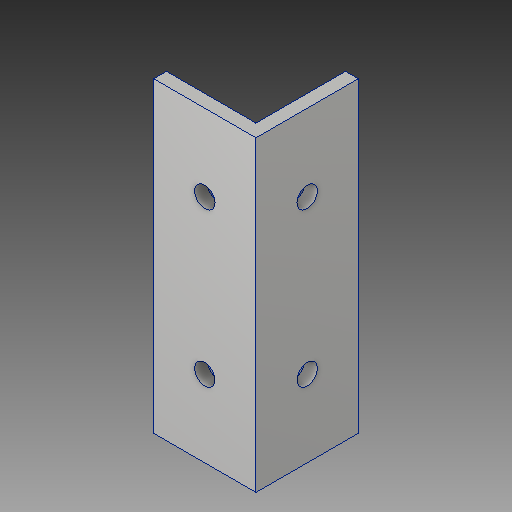
# Autodesk Inventor part: L Bracket 3in
Saved by Autodesk Inventor 2018 (Build 220112000, 112)
## iProperties
Created: 2018-01-19
Part Number: L Bracket 3in
Material: Aluminum 6061
Document SubType Name: Modeling
Designer: S-2512711
Density: 2.7 g/cm^3
Appearance: Aluminum - Flat
Mass: 30.4148 g
Surface Area: 80.8488 cm^2
Volume: 11.2647 cm^3
Author: S-2512711
Autodesk Inventor part; units mm, degrees
ref_plane "YZ Plane" through (0, 0, 0) normal (1, 0, 0) x (0, 1, 0)
ref_plane "XZ Plane" through (0, 0, 0) normal (0, 1, 0) x (-1, 0, 0)
ref_plane "XY Plane" through (0, 0, 0) normal (0, 0, 1) x (1, 0, 0)
sketch "Sketch1" plane through (0, 0, 0) normal (0, 1, 0) x (-1, 0, 0)
  line L0 (0, 0) -> (-25.4, 0)
  line L1 (-25.4, 0) -> (-25.4, -3.175)
  line L2 (-25.4, -3.175) -> (0, -3.175)
  line L3 (0, -3.175) -> (0, 0)
  line L4 (-25.4, 0) -> (-22.225, 0)
  line L5 (-22.225, 0) -> (-22.225, -25.4)
  line L6 (-22.225, -25.4) -> (-25.4, -25.4)
  line L7 (-25.4, -25.4) -> (-25.4, 0)
  dimension "d0" = 25.4
  dimension "d1" = 3.175
  dimension "d2" = 25.4
  dimension "d3" = 3.175
  constraints: 16 end point, 4 parallel, 2 horizontal, 2 perpendicular
  measures "d0" distance of L2.end L1.end
  measures "d1" distance of L5.end L6.end
  measures "d2" distance of L6.end L0.end
  measures "d3" distance of L2.end L0.start
extrude "Extrusion1" add sketch "Sketch1" along normal blind 76.2
sketch "Sketch2" plane through (25.4, 0, 0) normal (1, 0, 0) x (0, 0, -1)
  line L0 (0, 0) -> (0, 76.2) projected
  line L1 (0, 76.2) -> (12.7, 76.2)
  line L2 (12.7, 76.2) -> (12.7, 57.15)
  line L3 (0, 0) -> (25.4, 0) projected
  line L4 (12.7, 0) -> (12.7, 19.05)
  circle A0 centre (12.7, 57.15) radius 2.54
  circle A1 centre (12.7, 19.05) radius 2.54
  dimension "d6" = 12.7
  dimension "d7" = 19.05
  dimension "d8" = 19.05
  dimension "d9" = 5.08
  constraints: 6 end point, 2 centre point, 2 coincident, 1 horizontal, 1 midpoint, 1 perpendicular, 1 vertical
  measures "d6" distance of L0.end L1.end
  measures "d7" distance of L1.end L2.end
  measures "d8" distance of L4.start L4.end
  measures "d9" diameter of A0
extrude "Extrusion2" cut sketch "Sketch2" against normal blind 25.4
sketch "Sketch3" plane through (0, 0, 0) normal (0, 0, 1) x (1, 0, 0)
  line L0 (0, 0) -> (0, 76.2) projected
  line L1 (0, 76.2) -> (12.7, 76.2)
  line L2 (0, 76.2) -> (25.4, 76.2) projected
  line L3 (12.7, 76.2) -> (12.7, 57.15)
  line L4 (12.7, 0) -> (12.7, 19.05)
  circle A0 centre (12.7, 57.15) radius 2.54
  circle A1 centre (12.7, 19.05) radius 2.54
  dimension "d12" = 19.05
  dimension "d13" = 19.05
  dimension "d14" = 5.08
  constraints: 6 end point, 2 centre point, 2 coincident, 1 midpoint, 1 perpendicular, 1 vertical
  measures "d12" distance of L1.end L3.end
  measures "d13" distance of L4.start L4.end
  measures "d14" diameter of A0
extrude "Extrusion3" cut sketch "Sketch3" against normal blind 25.4
body "Solid1"
